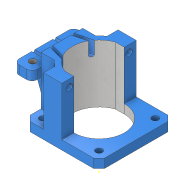
# Autodesk Inventor part: 7 peristaltic pump stator
Saved by Autodesk Inventor 2020 (Build 240168000, 168)
## iProperties
Created: 2018-08-21
Part Number: 7 peristaltic pump stator
Material: Generic
Document SubType Name: Modeling
Designer: mrbeh
Density: 1 g/cm^3
Appearance: Default
Author: mrbeh
Autodesk Inventor part; units mm, degrees
ref_plane "YZ Plane" through (0, 0, 0) normal (1, 0, 0) x (0, 1, 0)
ref_plane "XZ Plane" through (0, 0, 0) normal (0, 1, 0) x (-1, 0, 0)
sketch "Sketch1" plane through (0, 0, 0) normal (0, 1, 0) x (-1, 0, 0)
  line L0 (0, 0) -> (41, 0)
  line L1 (41, 0) -> (41, -41)
  line L2 (41, -41) -> (0, -41)
  line L3 (0, -41) -> (0, 0)
  dimension "d0" = 41
  dimension "d1" = 41
  constraints: 8 end point, 2 parallel, 1 horizontal, 1 perpendicular
  measures "d0" distance of L1.end L2.end
  measures "d1" distance of L0.end L1.end
extrude "Extrusion1" add sketch "Sketch1" along normal blind 5
sketch "Sketch2" plane through (0, 5, 0) normal (0, 1, 0) x (1, 0, 0)
  circle A0 centre (-20.5, 20.5) radius 7.5
  point P0 (0, 0)
  dimension "d4" = 15
  constraints: 1 centre point
  measures "d4" diameter of A0
extrude "Extrusion2" cut sketch "Sketch2" against normal blind 5
sketch "Sketch3" plane through (0, 5, 0) normal (0, 1, 0) x (1, 0, 0)
  circle A0 centre (-5, 5) radius 1.8
  point P0 (0, 0)
  dimension "d7" = 3.6
  constraints: 1 centre point
  measures "d7" diameter of A0
extrude "Extrusion3" cut sketch "Sketch3" against normal blind 5
pattern_linear "Rectangular Pattern1" count 2 spacing 31 along (0, 0, -1) count 2 spacing 31 along (-1, 0, 0) of "Extrusion3"
sketch "Sketch4" plane through (0, 5, 0) normal (0, 1, 0) x (1, 0, 0)
  circle A0 centre (-20.5, 20.5) radius 7.5 projected
  circle A1 centre (-20.5, 20.5) radius 12.15
  circle A2 centre (-20.5, 20.5) radius 17.5
  point P0 (0, 0)
  dimension "d16" = 24.3
  dimension "d17" = 35
  constraints: 2 centre point, 2 coincident
  measures "d16" diameter of A1
  measures "d17" diameter of A2
extrude "Extrusion4" add sketch "Sketch4" along normal blind 32 contours A2
sketch "Sketch5" plane through (-20.5, 37, -20.5) normal (0, 1, 0) x (1, 0, 0)
  line L0 (0, -23.8125) -> (19.05, -23.8125)
  line L1 (19.05, -23.8125) -> (19.05, 28.575)
  line L2 (19.05, 28.575) -> (0, 28.575)
  line L3 (0, 28.575) -> (0, -23.8125)
  point P0 (20.5, -20.5)
  constraints: 8 end point, 2 parallel, 1 horizontal, 1 perpendicular
extrude "Extrusion5" cut sketch "Sketch5" against normal blind 32
sketch "Sketch6" plane through (0, 37, 0) normal (0, 1, 0) x (1, 0, 0)
  arc A0 (-20.5, 32.65) -> (-20.5, 8.35) centre (-20.5, 20.5) ccw projected
  line L0 (0, 0) -> (-41, 0) projected
  line L1 (-20.5, 8.35) -> (-30.5, 8.35)
  line L2 (-30.5, 8.35) -> (-30.5, 0)
  line L3 (-30.5, 0) -> (-20.5, 0)
  line L4 (-20.5, 0) -> (-20.5, 8.35)
  dimension "d22" = 10
  constraints: 8 end point, 2 parallel, 1 horizontal, 1 perpendicular, 1 point on line
  measures "d22" distance of L3.end L2.end
extrude "Extrusion6" add sketch "Sketch6" against normal blind 32
ref_plane "Work Plane1" through (0, 0, -20.5) normal (0, 0, -1) x (-1, 0, 0)
mirror "Mirror1" about plane through (0, 0, -20.5) normal (0, 0, -1) of "Extrusion6"
sketch "Sketch8" plane through (0, 37, 0) normal (0, 1, 0) x (1, 0, 0)
  line L0 (-41, 41) -> (-41, 0) projected
  arc A0 (-30.5, 34.8614) -> (-30.5, 6.1386) centre (-20.5, 20.5) ccw projected
  line L1 (-41, 9) -> (-33.6909, 9)
  line L2 (-33.6909, 9) -> (-33.6909, 32)
  line L3 (-33.6909, 32) -> (-41, 32)
  line L4 (-41, 32) -> (-41, 9)
  point P0 (0, 0)
  dimension "d28" = 23
  constraints: 8 end point, 2 parallel, 1 horizontal, 1 perpendicular, 1 point on circle, 1 point on line
  measures "d28" distance of L2.end L1.end
extrude "Extrusion7" add sketch "Sketch8" against normal blind 32
sketch "Sketch9" plane through (0, 37, 0) normal (0, 1, 0) x (1, 0, 0)
  line L0 (-20.5, 41) -> (-20.5, 32.65) projected
  line L1 (-20.5, 32.65) -> (-41, 27.157)
  line L2 (-41, 0) -> (-41, 41) projected
  line L3 (-20.5, 32.65) -> (0.7232, 32.65) construction
  line L4 (-20.5, 30.9936) -> (-40.9092, 25.5249)
  line L5 (-40.9092, 25.5249) -> (-41.8751, 25.2661)
  line L6 (-40.9092, 25.5249) -> (-39.9092, 25.5249) construction
  line L7 (-41.8751, 25.2661) -> (-41, 27.157)
  line L8 (-20.5, 30.9936) -> (-20.5, 32.65)
  point P0 (0, 0)
  dimension "d31" = 165
  dimension "d32" = 1.6
  dimension "d33" = 1
  dimension "d34" = 165
  constraints: 14 end point, 2 equal length, 2 horizontal, 1 point on line, 1 vertical
  measures "d31" angle of L1 L3
  measures "d32" distance between parallel lines of L1 L4
  measures "d33" distance of L4.end L5.end
  measures "d34" angle of L5 L6
extrude "Extrusion8" cut sketch "Sketch9" against normal blind 7
mirror "Mirror2" about plane through (0, 0, -20.5) normal (0, 0, -1) of "Extrusion8"
sketch "Sketch10" plane through (-41, 0, -41) normal (-1, 0, 0) x (0, 0, 1)
  line L0 (27.157, 30) -> (25.5006, 30) projected
  circle A0 centre (26.3288, 30) radius 0.8282
  point P0 (41, 0)
  constraints: 1 horizontal alignment, 1 midpoint, 2 other
sketch "Sketch11" plane through (0, 37, 0) normal (0, 1, 0) x (1, 0, 0)
  line L0 (-41, 13.843) -> (-26.575, 9.9778) projected
  line L1 (-26.575, 9.9778) -> (-41, 13.843)
  point P0 (0, 0)
  constraints: 2 end point, 1 collinear
sketch3d "3D Sketch1"
  line L0 (-41, 37, -13.843) -> (-26.575, 37, -9.9778)
sweep "Sweep1" cut profiles "Sketch10" path "3D Sketch1"
mirror "Mirror3" about plane through (0, 0, -20.5) normal (0, 0, -1) of "Sweep1"
sketch "Sketch12" plane through (-41, 0, -41) normal (-1, 0, 0) x (0, 0, 1)
  line L0 (9, 5) -> (9, 37) projected
  line L1 (32, 30) -> (32, 25)
  line L2 (32, 25) -> (9, 25)
  line L3 (9, 25) -> (9, 30)
  arc A0 (13.843, 30) -> (15.4994, 30) centre (14.6712, 30) ccw projected
  arc A1 (13.843, 30) -> (15.4994, 30) centre (14.6712, 30) ccw
  arc A2 (25.5006, 30) -> (27.157, 30) centre (26.3288, 30) ccw projected
  arc A3 (25.5006, 30) -> (27.157, 30) centre (26.3288, 30) ccw
  line L4 (9, 30) -> (13.843, 30)
  line L5 (15.4994, 30) -> (25.5006, 30)
  line L6 (27.157, 30) -> (32, 30)
  point P0 (41, 0)
  dimension "d39" = 23
  dimension "d40" = 5
  constraints: 12 end point, 4 parallel, 4 point on circle, 3 horizontal, 3 perpendicular, 2 centre point, 2 coincident, 1 point on line
  measures "d39" distance of L1.end L2.end
  measures "d40" distance of L1.start L1.end
extrude "Extrusion9" add sketch "Sketch12" along normal blind 10
sketch "Sketch13" plane through (0, 5, 0) normal (0, 1, 0) x (1, 0, 0)
  circle A0 centre (-20.5, 20.5) radius 7.5 projected
  arc A1 (-20.5, 32.65) -> (-20.5, 8.35) centre (-20.5, 20.5) ccw projected
  circle A2 centre (-20.5, 20.5) radius 12.15
  point P0 (0, 0)
  constraints: 1 coincident, 1 vertical alignment, 2 other
extrude "Extrusion10" cut sketch "Sketch13" against normal blind 10
sketch "Sketch14" plane through (-41, 37, -9) normal (0, 0, 1) x (1, 0, 0)
  line L0 (0, -7) -> (-10, -7) projected
  line L1 (0, -12) -> (0, -32) projected
  line L2 (-10, -7) -> (0, -7)
  line L3 (0, -7) -> (0, -12)
  line L4 (0, -12) -> (-10, -12)
  line L5 (-10, -12) -> (-10, -7)
  point P0 (41, -37)
  constraints: 8 end point, 2 parallel, 1 horizontal, 1 perpendicular
extrude "Extrusion11" add sketch "Sketch14" along normal blind 5
mirror "Mirror4" about plane through (0, 0, -20.5) normal (0, 0, -1) of "Extrusion11"
sketch "Sketch15" plane through (-51, 30, -27.157) normal (0, 1, 0) x (1, 0, 0)
  circle A0 centre (5, 4.5) radius 1.8
  point P0 (51, -27.157)
  dimension "d81" = 3.6
  constraints: 1 centre point
  measures "d81" diameter of A0
extrude "Extrusion12" cut sketch "Sketch15" against normal blind 5
mirror "Mirror5" about plane through (0, 0, -20.5) normal (0, 0, -1) of "Extrusion12"
sketch "Sketch18" plane through (-51, 25, -4) normal (0, -1, 0) x (1, 0, 0)
  circle A0 centre (5, -27.657) radius 1.8 projected
  line L0 (7.8, -29.2736) -> (5, -30.8902)
  line L1 (5, -30.8902) -> (2.2, -29.2736)
  line L2 (2.2, -29.2736) -> (2.2, -26.0405)
  line L3 (2.2, -26.0405) -> (5, -24.4239)
  line L4 (5, -24.4239) -> (7.8, -26.0405)
  line L5 (7.8, -26.0405) -> (7.8, -29.2736)
  point P0 (51, 4)
  point P1 (4.5, -27.657)
  point P2 (4.5, -27.657)
  constraints: 12 end point, 2 coincident, 13 other
extrude "Extrusion14" cut sketch "Sketch18" against normal blind 2.5
mirror "Mirror6" about plane through (0, 0, -20.5) normal (0, 0, -1) of "Extrusion14"
sketch "Sketch19" plane through (-51, 25, -4) normal (0, -1, 0) x (1, 0, 0)
  line L0 (0, -22.5) -> (10, -22.5)
  line L1 (10, -22.5) -> (10, -10.5)
  line L2 (10, -10.5) -> (0, -10.5)
  line L3 (0, -10.5) -> (0, -22.5)
  line L4 (0, -22.5) -> (10, -10.5) construction
  line L5 (10, -22.5) -> (0, -10.5) construction
  point P0 (51, 4)
  point P1 (5, -16.5)
  dimension "d56" = 10
  dimension "d57" = 12
  constraints: 12 end point, 2 midpoint, 2 parallel, 1 horizontal, 1 perpendicular
  measures "d56" distance of L2.end L1.end
  measures "d57" distance of L1.end L0.end
extrude "Extrusion15" add sketch "Sketch19" along normal blind 25
chamfer "Chamfer1" distance 9 angle 70 1 edges at (-51, 0, -20.5) measured on face at (-50.5, 0, -20.5)
fillet "Fillet1" radius 3 4 edges at (-41, 27.5, -4) (-51, 27.5, -4) (-41, 27.5, -37) (-51, 27.5, -37)
sketch "Sketch20" plane through (-20.5, 37, 0) normal (1, 0, 0) x (0, 0, -1)
  circle A0 centre (4, -4) radius 1.8
  point P0 (0, -37)
  dimension "d64" = 3.6
  constraints: 1 centre point
  measures "d64" diameter of A0
extrude "Extrusion16" cut sketch "Sketch20" against normal blind 25
mirror "Mirror7" about plane through (0, 0, -20.5) normal (0, 0, -1) of "Extrusion16"
sketch "Sketch21" plane through (-30.5, 37, -41) normal (-1, 0, 0) x (0, 0, 1)
  circle A0 centre (4, -4) radius 1.8 projected
  line L0 (6.8, -5.6166) -> (4, -7.2332)
  line L1 (4, -7.2332) -> (1.2, -5.6166)
  line L2 (1.2, -5.6166) -> (1.2, -2.3834)
  line L3 (1.2, -2.3834) -> (4, -0.7668)
  line L4 (4, -0.7668) -> (6.8, -2.3834)
  line L5 (6.8, -2.3834) -> (6.8, -5.6166)
  point P0 (41, -37)
  constraints: 12 end point, 1 coincident, 13 other
extrude "Extrusion17" cut sketch "Sketch21" along normal blind 2.5 and the other way blind 2.5
mirror "Mirror8" about plane through (0, 0, -20.5) normal (0, 0, -1) of "Extrusion17"
chamfer "Chamfer2" distance 3 angle 45 4 edges at (-41, 2.5, 0) (-41, 2.5, -41) (0, 2.5, 0) (0, 2.5, -41)
thicken "Thicken1" operation add thickness 5 both sides no extend neighbours yes toward (0, 1, 0) faces at (-2.7833, 5, -20.5)
thicken "Thicken2" operation add thickness 5 both sides no extend neighbours yes toward (0, 1, 0) faces at (-34.6206, 5, -39.8943)
thicken "Thicken3" operation add thickness 5 both sides no extend neighbours yes toward (0, 1, 0) faces at (-34.6206, 5, -1.1057)
sketch "Sketch22" plane through (0, 0, 0) normal (0, -1, 0) x (1, 0, 0)
  line L0 (-61.9125, 0) -> (0, 0)
  line L1 (0, 0) -> (0, -47.625)
  line L2 (0, -47.625) -> (-61.9125, -47.625)
  line L3 (-61.9125, -47.625) -> (-61.9125, 0)
  constraints: 8 end point, 2 parallel, 1 horizontal, 1 perpendicular
extrude "Extrusion18" cut sketch "Sketch22" against normal blind 5
sketch "Sketch23" plane through (0, 5, 0) normal (0, -1, 0) x (1, 0, 0)
  point P0 (0, 0)
sketch "Sketch24" plane through (0, 5, 0) normal (0, -1, 0) x (1, 0, 0)
  arc A0 (-20.5, -32.65) -> (-20.5, -8.35) centre (-20.5, -20.5) ccw projected
  circle A1 centre (-20.5, -20.5) radius 14.7065
  point P0 (0, 0)
  dimension "d84" = 29.413
  constraints: 1 centre point, 1 coincident
  measures "d84" diameter of A1
extrude "Extrusion19" cut sketch "Sketch24" against normal blind 40
sketch "Sketch25" plane through (0, 37, 0) normal (0, 1, 0) x (1, 0, 0)
  arc A0 (-20.5, 5.7935) -> (-20.5, 35.2065) centre (-20.5, 20.5) ccw projected
  line L0 (-20.5, 5.7935) -> (-27.5, 5.7935)
  line L1 (-27.5, 5.7935) -> (-27.5, 6.5935)
  line L2 (-27.5, 6.5935) -> (-20.5, 6.5935)
  line L3 (-20.5, 6.5935) -> (-20.5, 5.7935)
  point P0 (0, 0)
  dimension "d87" = 7
  dimension "d88" = 0.8
  constraints: 8 end point, 2 parallel, 1 horizontal, 1 perpendicular
  measures "d87" distance of L1.end L2.end
  measures "d88" distance of L0.end L1.end
extrude "Extrusion20" add sketch "Sketch25" against normal up to surface (32 mm away)
mirror "Mirror9" about plane through (0, 0, -20.5) normal (0, 0, -1) of "Extrusion20"
thicken "Thicken4" operation add thickness 0.8 both sides no extend neighbours yes toward (-0.1604113, 0, 0.9870503) faces at (-18.1409, 6.6667, -35.0161)
body "Solid1"
